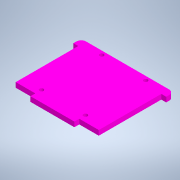
# Autodesk Inventor part: Bottom Base
Saved by Autodesk Inventor 2022 (Build 260153000, 153)
## iProperties
Created: 2021-07-09
Part Number: Bottom Base
Material: Generic
Document SubType Name: Modeling
Designer: benka
Density: 1 g/cm^3
Appearance: Magenta
Author: benka
Autodesk Inventor part; units mm, degrees
ref_plane "YZ Plane" through (0, 0, 0) normal (1, 0, 0) x (0, 1, 0)
ref_plane "XZ Plane" through (0, 0, 0) normal (0, 1, 0) x (-1, 0, 0)
ref_plane "XY Plane" through (0, 0, 0) normal (0, 0, 1) x (1, 0, 0)
sketch "Sketch1" plane through (22.5, 0, 39.0178) normal (0, 1, 0) x (-1, 0, 0)
  line L0 (0.0005, -5) -> (0.0005, 0)
  line L1 (45.0005, 0) -> (0.0005, 0)
  line L2 (45.0005, 0) -> (45.0005, -5)
  circle A0 centre (-0.0005, -73) radius 2
  circle A1 centre (0, -11.3502) radius 2
  circle A2 centre (45, -11.3502) radius 2
  circle A3 centre (44.9998, -73) radius 2
  line L3 (-20, -5) -> (0.0005, -5)
  line L4 (45.0005, -5) -> (65.0008, -5)
  line L5 (-20, -69) -> (-25.0002, -69)
  line L6 (-25.0002, -69) -> (-25.0002, -72)
  arc A4 (-25.0002, -72) -> (-20, -77) centre (-20.0002, -72) ccw
  line L7 (-20, -77) -> (65, -77)
  arc A5 (65, -77) -> (70, -72) centre (65, -72) ccw
  line L8 (70, -72) -> (70, -69)
  line L9 (70, -69) -> (64.9998, -69)
  line L10 (-20, -69) -> (-20, -5)
  line L11 (64.9998, -69) -> (65.0008, -5)
  point P0 (-25.0005, -77)
  point P1 (11.4357, -9.3722)
  dimension "d5" = 4
  dimension "d1" = 4
  dimension "d0" = 4
  constraints: 24 end point, 6 centre point, 4 point on circle
  measures "d5" diameter of A0
  measures "d1" diameter of A1
  measures "d0" diameter of A2
extrude "Bottom Base" add sketch "Sketch1" along normal blind 5
body "Solid1"
